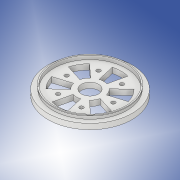
# Autodesk Inventor part: Flexspline
Saved by Autodesk Inventor 2017 SP1 (Build 210196100, 196)
## iProperties
Created: 2017-07-11
Part Number: Flexspline
Material: ABS Plastic
Document SubType Name: Modeling
Designer: zallen
Density: 1.06 g/cm^3
Appearance: CR White
Author: zallen
Autodesk Inventor part; units mm, degrees
ref_plane "YZ Plane" through (0, 0, 0) normal (1, 0, 0) x (0, 1, 0)
ref_plane "XZ Plane" through (0, 0, 0) normal (0, 1, 0) x (-1, 0, 0)
ref_plane "XY Plane" through (0, 0, 0) normal (0, 0, 1) x (1, 0, 0)
sketch "Sketch3" plane through (0, 0, 0) normal (0, 1, 0) x (-1, 0, 0)
  circle A0 centre (0, 0) radius 11
  circle A1 centre (0, 0) radius 17.5 construction
  circle A2 centre (0, 0) radius 40 construction
  circle A3 centre (0, 0) radius 54
  line L0 (-10, 38.7298) -> (-5, 16.7705)
  line L1 (10, 38.7298) -> (5, 16.7705)
  arc A4 (10, 38.7298) -> (-10, 38.7298) centre (0, 0) ccw
  arc A5 (5, 16.7705) -> (-5, 16.7705) centre (0, 0) ccw
  circle A6 centre (0, 0) radius 30 construction
  line L2 (7.7787, 28.974) -> (21.2029, 21.2235) construction
  line L3 (14.4908, 25.0988) -> (15, 25.9808) construction
  circle A7 centre (15, 25.9808) radius 2.5
  circle A8 centre (-15, 25.9808) radius 2.5
  circle A9 centre (-30, 0) radius 2.5
  circle A10 centre (-15, -25.9808) radius 2.5
  circle A11 centre (15, -25.9808) radius 2.5
  circle A12 centre (30, 0) radius 2.5
  arc A13 (-28.541, 28.0252) -> (-38.541, 10.7047) centre (0, 0) ccw
  line L4 (-28.541, 28.0252) -> (-12.0237, 12.7154)
  line L5 (-38.541, 10.7047) -> (-17.0237, 4.0551)
  arc A14 (-12.0237, 12.7154) -> (-17.0237, 4.0551) centre (0, 0) ccw
  arc A15 (-38.541, -10.7047) -> (-28.541, -28.0252) centre (0, 0) ccw
  line L6 (-38.541, -10.7047) -> (-17.0237, -4.0551)
  line L7 (-28.541, -28.0252) -> (-12.0237, -12.7154)
  arc A16 (-17.0237, -4.0551) -> (-12.0237, -12.7154) centre (0, 0) ccw
  arc A17 (-10, -38.7298) -> (10, -38.7298) centre (0, 0) ccw
  line L8 (-10, -38.7298) -> (-5, -16.7705)
  line L9 (10, -38.7298) -> (5, -16.7705)
  arc A18 (-5, -16.7705) -> (5, -16.7705) centre (0, 0) ccw
  arc A19 (28.541, -28.0252) -> (38.541, -10.7047) centre (0, 0) ccw
  line L10 (28.541, -28.0252) -> (12.0237, -12.7154)
  line L11 (38.541, -10.7047) -> (17.0237, -4.0551)
  arc A20 (12.0237, -12.7154) -> (17.0237, -4.0551) centre (0, 0) ccw
  arc A21 (38.541, 10.7047) -> (28.541, 28.0252) centre (0, 0) ccw
  line L12 (38.541, 10.7047) -> (17.0237, 4.0551)
  line L13 (28.541, 28.0252) -> (12.0237, 12.7154)
  arc A22 (17.0237, 4.0551) -> (12.0237, 12.7154) centre (0, 0) ccw
  point P0 (-21.2029, 21.2235)
  point P1 (-28.9815, -7.7505)
  point P2 (-7.7787, -28.974)
  point P3 (21.2029, -21.2235)
  point P4 (28.9815, 7.7505)
  dimension "d16" = 22
  dimension "d17" = 35
  dimension "d18" = 80
  dimension "d19" = 108
  dimension "d20" = 10
  dimension "d21" = 5
  dimension "d22" = 10
  dimension "d23" = 5
  dimension "d28" = 60
  dimension "d29" = 5
  dimension "d32" = 360
  dimension "d38" = 360
  constraints: 31 point on circle, 28 end point, 23 centre point, 7 point on line, 6 coincident, 3 concentric, 1 midpoint, 1 perpendicular, 80 other
  measures "d16" diameter of A0
  measures "d17" diameter of A1
  measures "d18" diameter of A2
  measures "d19" diameter of A3
  measures "d20" horizontal distance of point (0, 0) L0.start
  measures "d21" horizontal distance of point (0, 0) L0.end
  measures "d22" horizontal distance of point (0, 0) L1.start
  measures "d23" horizontal distance of point (0, 0) L1.end
  measures "d28" diameter of A6
  measures "d29" diameter of A7
extrude "Extrusion4" add sketch "Sketch3" along normal blind 7
sketch "Sketch4" plane through (0, 7, 0) normal (0, 1, 0) x (1, 0, 0)
  circle A0 centre (0, 0) radius 47.5
  circle A1 centre (0, 0) radius 46.5
  dimension "d42" = 95
  dimension "d43" = 93
  constraints: 2 centre point, 2 coincident
  measures "d42" diameter of A0
  measures "d43" diameter of A1
extrude "Extrusion5" add sketch "Sketch4" along normal blind 4
sketch "Sketch6" plane through (0, 11, 0) normal (0, 1, 0) x (1, 0, 0)
  circle A0 centre (0, 0) radius 46.5 projected
  circle A1 centre (0, 0) radius 48
  dimension "d49" = 96
  constraints: 1 centre point, 1 coincident
  measures "d49" diameter of A1
extrude "Extrusion7" add sketch "Sketch6" along normal blind 1
body "Solid1"
